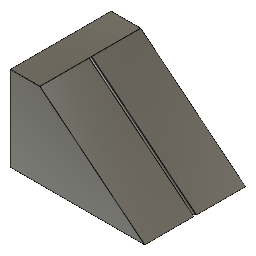
angled tube holder v6 (Autodesk Fusion 360 design; units mm, degrees)
Autodesk Fusion 360 part; units mm, degrees
sketch "side profile" plane through (0, 0, 0) normal (0, 1, 0) x (1, 0, 0)
  line L0 (0, 0) -> (80, 0)
  line L1 (80, 0) -> (17.6527, -50.4606)
  line L2 (17.6527, -50.4606) -> (0, -50.4606)
  line L3 (0, -50.4606) -> (0, 0)
  dimension "d1" = 80.2088
  dimension "d2" = 38.985
  dimension "d3" = 80
  constraint coincident L0.start L3.end
  constraint horizontal L0
  constraint perpendicular L0 L3
  constraint horizontal L2
  measures "d1" distance of L0.end L1.end
  measures "d2" angle of L0 L1
  measures "d3" distance of L0.start L0.end
extrude "Extrude1" add sketch "side profile" along normal blind 60
sketch "tube holder" plane through (31.6629, 0, 39.1215) normal (0.629115, 0, 0.777312) x (0, 1, 0)
  line L0 (0, 18.0239) -> (0, -62.185)
  line L1 (0, -62.185) -> (60, -62.185)
  line L2 (60, -62.185) -> (60, 18.0239)
  line L3 (60, 18.0239) -> (0, 18.0239)
  line L4 (30, 18.0239) -> (30, -62.185)
  constraint midpoint L3 L4.start
  constraint midpoint L1 L4.end
pipe "Pipe1" cut diameter 1.5 path "tube holder" along L4
